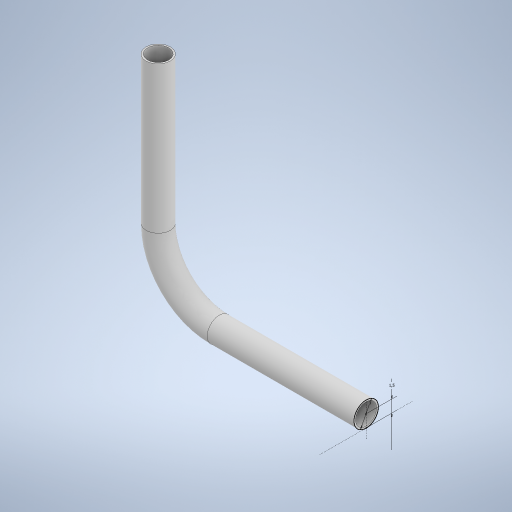
# Autodesk Inventor part: Hudson 1-70
Saved by Autodesk Inventor 2024.2 (Build 282272000, 272)
## iProperties
Created: 2024-10-10
Part Number: Hudson 1-70
Material: Generic
Document SubType Name: Modeling
Designer: Precisión-12
Density: 1 g/cm^3
Appearance: Default
Author: Precisión-12
Autodesk Inventor part; units mm, degrees
ref_plane "YZ Plane" through (0, 0, 0) normal (1, 0, 0) x (0, 1, 0)
ref_plane "XY Plane" through (0, 0, 0) normal (0, 0, 1) x (1, 0, 0)
sketch "Sketch1" plane through (0, 0, 0) normal (0, 0, 1) x (1, 0, 0)
  line L0 (0, 0) -> (-27, 0)
  line L1 (-27, 0) -> (-27, 27)
  arc A0 (-24, 9) -> (-18, 3) centre (-18, 9) ccw
  arc A1 (-27, 9) -> (-18, 0) centre (-18, 9) ccw
  line L2 (0, 3) -> (-18, 3)
  line L3 (-24, 9) -> (-24, 27)
  line L4 (0, 0) -> (0, 3)
  line L5 (-27, 27) -> (-24, 27)
  line L6 (-25.5, 9) -> (-25.5, 27)
  line L7 (-18, 1.5) -> (0, 1.5)
  arc A2 (-25.5, 9) -> (-18, 1.5) centre (-18, 9) ccw
  line L8 (-24, 9) -> (-27, 9)
  line L9 (-18, 3) -> (-18, 0)
  dimension "d0" = 27
  dimension "d1" = 27
  dimension "d2" = 6
  dimension "d3" = 9
  constraints: 20 end point, 7 point on circle, 5 tangent, 4 perpendicular, 3 centre point, 2 horizontal, 2 midpoint, 2 point on line, 1 coincident, 1 parallel, 1 vertical
  measures "d0" distance of L0.start L0.end
  measures "d1" distance of L0.end L1.end
  measures "d2" radius of A0
  measures "d3" radius of A1
sketch "Sketch2" plane through (0, 0, 0) normal (1, 0, 0) x (0, 1, 0)
  circle A0 centre (1.5, 0) radius 1.5
  line L0 (0, 5.6966) -> (0, -5.6966) construction
  line L1 (3, 0) -> (-1.1636, 0) construction
  point P0 (0, 0)
  point P1 (0, 0)
  dimension "d5" = 3
  dimension "d6" = 1.5
  constraints: 4 end point, 2 point on line, 1 coincident, 1 horizontal, 1 horizontal alignment, 1 midpoint, 1 vertical, 2 other
  measures "d6" distance of point (0, 0) point (1.5, 0)
ref_plane "Work Plane1" through (0, 27, 0) normal (0, 1, 0) x (-1, 0, 0)
sketch "Sketch3" plane through (0, 27, 0) normal (0, 1, 0) x (-1, 0, 0)
  circle A0 centre (25.5, 0) radius 1.5
  line L0 (27, 6.8213) -> (27, -6.8213) construction
  line L1 (30.5412, 0) -> (-1.145, 0) construction
  point P0 (0, 0)
  point P1 (27, 0)
  dimension "d8" = 3
  dimension "d9" = 27
  dimension "d10" = 25.5
  constraints: 4 end point, 3 point on line, 1 centre point, 1 horizontal, 1 midpoint, 1 vertical
  measures "d8" diameter of A0
  measures "d9" distance from line of point (0, 0) L0
  measures "d10" distance of point (0, 0) A0.centre
sweep "Sweep1" add profiles "Sketch3" path "Sketch1" path curves L6 A2 L7
shell "Shell1" thickness 0.2 removed faces 2 at (0, 1.8952, 0.8627) at (-25.3633, 27, 0.3027)
body "Solid1"
